Autodesk Fusion 360 part; units mm, degrees
(part 2 of 5)
sketch "Top Projection" plane through (0, 0, 0) normal (0, 0, 1) x (1, 0, 0) in component "Top"
  line L0 (0, 16.095) -> (-1.5613, 16.095)
  arc A0 (-3.175, 17.2242) -> (-1.5613, 16.095) centre (-2.4679, 16.5171) ccw
  line L1 (-3.175, 17.2242) -> (-3.175, 24.7758)
  arc A1 (-1.5613, 25.905) -> (-3.175, 24.7758) centre (-2.4679, 25.4829) ccw
  line L2 (-1.5613, 25.905) -> (0, 25.905)
  line L3 (0, 25.905) -> (0, 36.095)
  line L4 (0, 36.095) -> (-1.5613, 36.095)
  arc A2 (-3.175, 37.2242) -> (-1.5613, 36.095) centre (-2.4679, 36.5171) ccw
  line L5 (-3.175, 37.2242) -> (-3.175, 44.7758)
  arc A3 (-1.5613, 45.905) -> (-3.175, 44.7758) centre (-2.4679, 45.4829) ccw
  line L6 (-1.5613, 45.905) -> (0, 45.905)
  line L7 (0, 45.905) -> (0, 56.095)
  line L8 (0, 56.095) -> (-1.5613, 56.095)
  arc A4 (-3.175, 57.2242) -> (-1.5613, 56.095) centre (-2.4679, 56.5171) ccw
  line L9 (-3.175, 57.2242) -> (-3.175, 64.7758)
  arc A5 (-1.5613, 65.905) -> (-3.175, 64.7758) centre (-2.4679, 65.4829) ccw
  line L10 (-1.5613, 65.905) -> (0, 65.905)
  line L11 (0, 65.905) -> (0, 76.095)
  line L12 (0, 76.095) -> (-1.5613, 76.095)
  arc A6 (-3.175, 77.2242) -> (-1.5613, 76.095) centre (-2.4679, 76.5171) ccw
  line L13 (-3.175, 77.2242) -> (-3.175, 84.7758)
  arc A7 (-1.5613, 85.905) -> (-3.175, 84.7758) centre (-2.4679, 85.4829) ccw
  line L14 (-1.5613, 85.905) -> (0, 85.905)
  line L15 (0, 85.905) -> (0, 96.095)
  line L16 (0, 96.095) -> (-1.5613, 96.095)
  arc A8 (-3.175, 97.2242) -> (-1.5613, 96.095) centre (-2.4679, 96.5171) ccw
  line L17 (-3.175, 97.2242) -> (-3.175, 104.7758)
  arc A9 (-1.5613, 105.905) -> (-3.175, 104.7758) centre (-2.4679, 105.4829) ccw
  line L18 (-1.5613, 105.905) -> (0, 105.905)
  line L19 (0, 105.905) -> (0, 116.095)
  line L20 (0, 116.095) -> (-1.5613, 116.095)
  arc A10 (-3.175, 117.2242) -> (-1.5613, 116.095) centre (-2.4679, 116.5171) ccw
  line L21 (-3.175, 117.2242) -> (-3.175, 124.7758)
  arc A11 (-1.5613, 125.905) -> (-3.175, 124.7758) centre (-2.4679, 125.4829) ccw
  line L22 (-1.5613, 125.905) -> (0, 125.905)
  line L23 (0, 125.905) -> (0, 136.095)
  line L24 (0, 136.095) -> (-1.5613, 136.095)
  arc A12 (-3.175, 137.2242) -> (-1.5613, 136.095) centre (-2.4679, 136.5171) ccw
  line L25 (-3.175, 137.2242) -> (-3.175, 144.7758)
  arc A13 (-1.5613, 145.905) -> (-3.175, 144.7758) centre (-2.4679, 145.4829) ccw
  line L26 (-1.5613, 145.905) -> (0, 145.905)
  line L27 (0, 145.905) -> (0, 156.095)
  line L28 (0, 156.095) -> (-1.5613, 156.095)
  arc A14 (-3.175, 157.2242) -> (-1.5613, 156.095) centre (-2.4679, 156.5171) ccw
  line L29 (-3.175, 157.2242) -> (-3.175, 164.7758)
  arc A15 (-1.5613, 165.905) -> (-3.175, 164.7758) centre (-2.4679, 165.4829) ccw
  line L30 (-1.5613, 165.905) -> (0, 165.905)
  line L31 (0, 165.905) -> (0, 182)
  line L32 (0, 182) -> (-15.095, 182)
  line L33 (-240, 182) -> (-240, 165.905)
  line L34 (-240, 165.905) -> (-238.4387, 165.905)
  arc A16 (-236.825, 164.7758) -> (-238.4387, 165.905) centre (-237.5321, 165.4829) ccw
  line L35 (-236.825, 164.7758) -> (-236.825, 157.2242)
  arc A17 (-238.4387, 156.095) -> (-236.825, 157.2242) centre (-237.5321, 156.5171) ccw
  line L36 (-238.4387, 156.095) -> (-240, 156.095)
  line L37 (-240, 156.095) -> (-240, 145.905)
  line L38 (-240, 145.905) -> (-238.4387, 145.905)
  arc A18 (-236.825, 144.7758) -> (-238.4387, 145.905) centre (-237.5321, 145.4829) ccw
  line L39 (-236.825, 144.7758) -> (-236.825, 137.2242)
  arc A19 (-238.4387, 136.095) -> (-236.825, 137.2242) centre (-237.5321, 136.5171) ccw
  line L40 (-238.4387, 136.095) -> (-240, 136.095)
  line L41 (-240, 136.095) -> (-240, 125.905)
  line L42 (-240, 125.905) -> (-238.4387, 125.905)
  arc A20 (-236.825, 124.7758) -> (-238.4387, 125.905) centre (-237.5321, 125.4829) ccw
  line L43 (-236.825, 124.7758) -> (-236.825, 117.2242)
  arc A21 (-238.4387, 116.095) -> (-236.825, 117.2242) centre (-237.5321, 116.5171) ccw
  line L44 (-238.4387, 116.095) -> (-240, 116.095)
  line L45 (-240, 116.095) -> (-240, 105.905)
  line L46 (-240, 105.905) -> (-238.4387, 105.905)
  arc A22 (-236.825, 104.7758) -> (-238.4387, 105.905) centre (-237.5321, 105.4829) ccw
  line L47 (-236.825, 104.7758) -> (-236.825, 97.2242)
  arc A23 (-238.4387, 96.095) -> (-236.825, 97.2242) centre (-237.5321, 96.5171) ccw
  line L48 (-238.4387, 96.095) -> (-240, 96.095)
  line L49 (-240, 96.095) -> (-240, 85.905)
  line L50 (-240, 85.905) -> (-238.4387, 85.905)
  arc A24 (-236.825, 84.7758) -> (-238.4387, 85.905) centre (-237.5321, 85.4829) ccw
  line L51 (-236.825, 84.7758) -> (-236.825, 77.2242)
  arc A25 (-238.4387, 76.095) -> (-236.825, 77.2242) centre (-237.5321, 76.5171) ccw
  line L52 (-238.4387, 76.095) -> (-240, 76.095)
  line L53 (-240, 76.095) -> (-240, 65.905)
  line L54 (-240, 65.905) -> (-238.4387, 65.905)
  arc A26 (-236.825, 64.7758) -> (-238.4387, 65.905) centre (-237.5321, 65.4829) ccw
  line L55 (-236.825, 64.7758) -> (-236.825, 57.2242)
  arc A27 (-238.4387, 56.095) -> (-236.825, 57.2242) centre (-237.5321, 56.5171) ccw
  line L56 (-238.4387, 56.095) -> (-240, 56.095)
  line L57 (-240, 56.095) -> (-240, 45.905)
  line L58 (-240, 45.905) -> (-238.4387, 45.905)
  arc A28 (-236.825, 44.7758) -> (-238.4387, 45.905) centre (-237.5321, 45.4829) ccw
  line L59 (-236.825, 44.7758) -> (-236.825, 37.2242)
  arc A29 (-238.4387, 36.095) -> (-236.825, 37.2242) centre (-237.5321, 36.5171) ccw
  line L60 (-238.4387, 36.095) -> (-240, 36.095)
  line L61 (-240, 36.095) -> (-240, 25.905)
  line L62 (-240, 25.905) -> (-238.4387, 25.905)
  arc A30 (-236.825, 24.7758) -> (-238.4387, 25.905) centre (-237.5321, 25.4829) ccw
  line L63 (-236.825, 24.7758) -> (-236.825, 17.2242)
  arc A31 (-238.4387, 16.095) -> (-236.825, 17.2242) centre (-237.5321, 16.5171) ccw
  line L64 (-238.4387, 16.095) -> (-240, 16.095)
  line L65 (-240, 16.095) -> (-240, 0)
  line L66 (-240, 0) -> (-224.905, 0)
  line L67 (-224.905, 0) -> (-224.905, 1.5613)
  arc A32 (-223.7758, 3.175) -> (-224.905, 1.5613) centre (-224.4829, 2.4679) ccw
  line L68 (-223.7758, 3.175) -> (-216.2242, 3.175)
  arc A33 (-215.095, 1.5613) -> (-216.2242, 3.175) centre (-215.5171, 2.4679) ccw
  line L69 (-215.095, 1.5613) -> (-215.095, 0)
  line L70 (-215.095, 0) -> (-204.905, 0)
  line L71 (-204.905, 0) -> (-204.905, 1.5613)
  arc A34 (-203.7758, 3.175) -> (-204.905, 1.5613) centre (-204.4829, 2.4679) ccw
  line L72 (-203.7758, 3.175) -> (-196.2242, 3.175)
  arc A35 (-195.095, 1.5613) -> (-196.2242, 3.175) centre (-195.5171, 2.4679) ccw
  line L73 (-195.095, 1.5613) -> (-195.095, 0)
  line L74 (-195.095, 0) -> (-184.905, 0)
  line L75 (-184.905, 0) -> (-184.905, 1.5613)
  arc A36 (-183.7758, 3.175) -> (-184.905, 1.5613) centre (-184.4829, 2.4679) ccw
  line L76 (-183.7758, 3.175) -> (-176.2242, 3.175)
  arc A37 (-175.095, 1.5613) -> (-176.2242, 3.175) centre (-175.5171, 2.4679) ccw
  line L77 (-175.095, 1.5613) -> (-175.095, 0)
  line L78 (-175.095, 0) -> (-164.905, 0)
  line L79 (-164.905, 0) -> (-164.905, 1.5613)
  arc A38 (-163.7758, 3.175) -> (-164.905, 1.5613) centre (-164.4829, 2.4679) ccw
  line L80 (-163.7758, 3.175) -> (-156.2242, 3.175)
  arc A39 (-155.095, 1.5613) -> (-156.2242, 3.175) centre (-155.5171, 2.4679) ccw
  line L81 (-155.095, 1.5613) -> (-155.095, 0)
  line L82 (-155.095, 0) -> (-144.905, 0)
  line L83 (-144.905, 0) -> (-144.905, 1.5613)
  arc A40 (-143.7758, 3.175) -> (-144.905, 1.5613) centre (-144.4829, 2.4679) ccw
  line L84 (-143.7758, 3.175) -> (-136.2242, 3.175)
  arc A41 (-135.095, 1.5613) -> (-136.2242, 3.175) centre (-135.5171, 2.4679) ccw
  line L85 (-135.095, 1.5613) -> (-135.095, 0)
  line L86 (-135.095, 0) -> (-124.905, 0)
  line L87 (-124.905, 0) -> (-124.905, 1.5613)
  arc A42 (-123.7758, 3.175) -> (-124.905, 1.5613) centre (-124.4829, 2.4679) ccw
  line L88 (-123.7758, 3.175) -> (-116.2242, 3.175)
  arc A43 (-115.095, 1.5613) -> (-116.2242, 3.175) centre (-115.5171, 2.4679) ccw
  line L89 (-115.095, 1.5613) -> (-115.095, 0)
  line L90 (-115.095, 0) -> (-104.905, 0)
  line L91 (-104.905, 0) -> (-104.905, 1.5613)
  arc A44 (-103.7758, 3.175) -> (-104.905, 1.5613) centre (-104.4829, 2.4679) ccw
  line L92 (-103.7758, 3.175) -> (-96.2242, 3.175)
  arc A45 (-95.095, 1.5613) -> (-96.2242, 3.175) centre (-95.5171, 2.4679) ccw
  line L93 (-95.095, 1.5613) -> (-95.095, 0)
  line L94 (-95.095, 0) -> (-84.905, 0)
  line L95 (-84.905, 0) -> (-84.905, 1.5613)
  arc A46 (-83.7758, 3.175) -> (-84.905, 1.5613) centre (-84.4829, 2.4679) ccw
  line L96 (-83.7758, 3.175) -> (-76.2242, 3.175)
  arc A47 (-75.095, 1.5613) -> (-76.2242, 3.175) centre (-75.5171, 2.4679) ccw
  line L97 (-75.095, 1.5613) -> (-75.095, 0)
  line L98 (-75.095, 0) -> (-64.905, 0)
  line L99 (-64.905, 0) -> (-64.905, 1.5613)
  arc A48 (-63.7758, 3.175) -> (-64.905, 1.5613) centre (-64.4829, 2.4679) ccw
  line L100 (-63.7758, 3.175) -> (-56.2242, 3.175)
  arc A49 (-55.095, 1.5613) -> (-56.2242, 3.175) centre (-55.5171, 2.4679) ccw
  line L101 (-55.095, 1.5613) -> (-55.095, 0)
  line L102 (-55.095, 0) -> (-44.905, 0)
  line L103 (-44.905, 0) -> (-44.905, 1.5613)
  arc A50 (-43.7758, 3.175) -> (-44.905, 1.5613) centre (-44.4829, 2.4679) ccw
  line L104 (-43.7758, 3.175) -> (-36.2242, 3.175)
  arc A51 (-35.095, 1.5613) -> (-36.2242, 3.175) centre (-35.5171, 2.4679) ccw
  line L105 (-35.095, 1.5613) -> (-35.095, 0)
  line L106 (-35.095, 0) -> (-24.905, 0)
  line L107 (-24.905, 0) -> (-24.905, 1.5613)
  arc A52 (-23.7758, 3.175) -> (-24.905, 1.5613) centre (-24.4829, 2.4679) ccw
  line L108 (-23.7758, 3.175) -> (-16.2242, 3.175)
  arc A53 (-15.095, 1.5613) -> (-16.2242, 3.175) centre (-15.5171, 2.4679) ccw
  line L109 (-15.095, 1.5613) -> (-15.095, 0)
  line L110 (-15.095, 0) -> (0, 0)
  line L111 (0, 0) -> (0, 16.095)
  line L112 (-15.095, 182) -> (-15.095, 180.4387)
  arc A54 (-16.2242, 178.825) -> (-15.095, 180.4387) centre (-15.5171, 179.5321) ccw
  line L113 (-16.2242, 178.825) -> (-23.7758, 178.825)
  arc A55 (-24.905, 180.4387) -> (-23.7758, 178.825) centre (-24.4829, 179.5321) ccw
  line L114 (-24.905, 180.4387) -> (-24.905, 182)
  line L115 (-24.905, 182) -> (-35.095, 182)
  line L116 (-35.095, 182) -> (-35.095, 180.4387)
  arc A56 (-36.2242, 178.825) -> (-35.095, 180.4387) centre (-35.5171, 179.5321) ccw
  line L117 (-36.2242, 178.825) -> (-43.7758, 178.825)
  arc A57 (-44.905, 180.4387) -> (-43.7758, 178.825) centre (-44.4829, 179.5321) ccw
  line L118 (-44.905, 180.4387) -> (-44.905, 182)
  line L119 (-44.905, 182) -> (-55.095, 182)
  line L120 (-55.095, 182) -> (-55.095, 180.4387)
  arc A58 (-56.2242, 178.825) -> (-55.095, 180.4387) centre (-55.5171, 179.5321) ccw
  line L121 (-56.2242, 178.825) -> (-63.7758, 178.825)
  arc A59 (-64.905, 180.4387) -> (-63.7758, 178.825) centre (-64.4829, 179.5321) ccw
  line L122 (-64.905, 180.4387) -> (-64.905, 182)
  line L123 (-64.905, 182) -> (-75.095, 182)
  line L124 (-75.095, 182) -> (-75.095, 180.4387)
  arc A60 (-76.2242, 178.825) -> (-75.095, 180.4387) centre (-75.5171, 179.5321) ccw
  line L125 (-76.2242, 178.825) -> (-83.7758, 178.825)
  arc A61 (-84.905, 180.4387) -> (-83.7758, 178.825) centre (-84.4829, 179.5321) ccw
  line L126 (-84.905, 180.4387) -> (-84.905, 182)
  line L127 (-84.905, 182) -> (-95.095, 182)
  line L128 (-95.095, 182) -> (-95.095, 180.4387)
  arc A62 (-96.2242, 178.825) -> (-95.095, 180.4387) centre (-95.5171, 179.5321) ccw
  line L129 (-96.2242, 178.825) -> (-103.7758, 178.825)
  arc A63 (-104.905, 180.4387) -> (-103.7758, 178.825) centre (-104.4829, 179.5321) ccw
  line L130 (-104.905, 180.4387) -> (-104.905, 182)
  line L131 (-104.905, 182) -> (-115.095, 182)
  line L132 (-115.095, 182) -> (-115.095, 180.4387)
  arc A64 (-116.2242, 178.825) -> (-115.095, 180.4387) centre (-115.5171, 179.5321) ccw
  line L133 (-116.2242, 178.825) -> (-123.7758, 178.825)
  arc A65 (-124.905, 180.4387) -> (-123.7758, 178.825) centre (-124.4829, 179.5321) ccw
  line L134 (-124.905, 180.4387) -> (-124.905, 182)
  line L135 (-124.905, 182) -> (-135.095, 182)
  line L136 (-135.095, 182) -> (-135.095, 180.4387)
  arc A66 (-136.2242, 178.825) -> (-135.095, 180.4387) centre (-135.5171, 179.5321) ccw
  line L137 (-136.2242, 178.825) -> (-143.7758, 178.825)
  arc A67 (-144.905, 180.4387) -> (-143.7758, 178.825) centre (-144.4829, 179.5321) ccw
  line L138 (-144.905, 180.4387) -> (-144.905, 182)
  line L139 (-144.905, 182) -> (-155.095, 182)
  line L140 (-155.095, 182) -> (-155.095, 180.4387)
  arc A68 (-156.2242, 178.825) -> (-155.095, 180.4387) centre (-155.5171, 179.5321) ccw
  line L141 (-156.2242, 178.825) -> (-163.7758, 178.825)
  arc A69 (-164.905, 180.4387) -> (-163.7758, 178.825) centre (-164.4829, 179.5321) ccw
  line L142 (-164.905, 180.4387) -> (-164.905, 182)
  line L143 (-164.905, 182) -> (-175.095, 182)
  line L144 (-175.095, 182) -> (-175.095, 180.4387)
  arc A70 (-176.2242, 178.825) -> (-175.095, 180.4387) centre (-175.5171, 179.5321) ccw
  line L145 (-176.2242, 178.825) -> (-183.7758, 178.825)
  arc A71 (-184.905, 180.4387) -> (-183.7758, 178.825) centre (-184.4829, 179.5321) ccw
  line L146 (-184.905, 180.4387) -> (-184.905, 182)
  line L147 (-184.905, 182) -> (-195.095, 182)
  line L148 (-195.095, 182) -> (-195.095, 180.4387)
  arc A72 (-196.2242, 178.825) -> (-195.095, 180.4387) centre (-195.5171, 179.5321) ccw
  line L149 (-196.2242, 178.825) -> (-203.7758, 178.825)
  arc A73 (-204.905, 180.4387) -> (-203.7758, 178.825) centre (-204.4829, 179.5321) ccw
  line L150 (-204.905, 180.4387) -> (-204.905, 182)
  line L151 (-204.905, 182) -> (-215.095, 182)
  line L152 (-215.095, 182) -> (-215.095, 180.4387)
  arc A74 (-216.2242, 178.825) -> (-215.095, 180.4387) centre (-215.5171, 179.5321) ccw
  line L153 (-216.2242, 178.825) -> (-223.7758, 178.825)
  arc A75 (-224.905, 180.4387) -> (-223.7758, 178.825) centre (-224.4829, 179.5321) ccw
  line L154 (-224.905, 180.4387) -> (-224.905, 182)
  line L155 (-224.905, 182) -> (-240, 182)
sketch "Bottom Projection" plane through (0, 0, 0) normal (0, 0, 1) x (1, 0, 0) in component "Bottom"
  line L0 (0, -158.095) -> (-1.5613, -158.095)
  arc A0 (-1.5613, -158.095) -> (-3.175, -159.2242) centre (-2.4679, -158.5171) ccw
  line L1 (-3.175, -159.2242) -> (-3.175, -166.7758)
  arc A1 (-3.175, -166.7758) -> (-1.5613, -167.905) centre (-2.4679, -167.4829) ccw
  line L2 (-1.5613, -167.905) -> (0, -167.905)
  line L3 (0, -138.095) -> (-1.5613, -138.095)
  arc A2 (-1.5613, -138.095) -> (-3.175, -139.2242) centre (-2.4679, -138.5171) ccw
  line L4 (-3.175, -139.2242) -> (-3.175, -146.7758)
  arc A3 (-3.175, -146.7758) -> (-1.5613, -147.905) centre (-2.4679, -147.4829) ccw
  line L5 (-1.5613, -147.905) -> (0, -147.905)
  line L6 (0, -118.095) -> (-1.5613, -118.095)
  arc A4 (-1.5613, -118.095) -> (-3.175, -119.2242) centre (-2.4679, -118.5171) ccw
  line L7 (-3.175, -119.2242) -> (-3.175, -126.7758)
  arc A5 (-3.175, -126.7758) -> (-1.5613, -127.905) centre (-2.4679, -127.4829) ccw
  line L8 (-1.5613, -127.905) -> (0, -127.905)
  line L9 (0, -98.095) -> (-1.5613, -98.095)
  arc A6 (-1.5613, -98.095) -> (-3.175, -99.2242) centre (-2.4679, -98.5171) ccw
  line L10 (-3.175, -99.2242) -> (-3.175, -106.7758)
  arc A7 (-3.175, -106.7758) -> (-1.5613, -107.905) centre (-2.4679, -107.4829) ccw
  line L11 (-1.5613, -107.905) -> (0, -107.905)
  line L12 (0, -78.095) -> (-1.5613, -78.095)
  arc A8 (-1.5613, -78.095) -> (-3.175, -79.2242) centre (-2.4679, -78.5171) ccw
  line L13 (-3.175, -79.2242) -> (-3.175, -86.7758)
  arc A9 (-3.175, -86.7758) -> (-1.5613, -87.905) centre (-2.4679, -87.4829) ccw
  line L14 (-1.5613, -87.905) -> (0, -87.905)
  line L15 (0, -58.095) -> (-1.5613, -58.095)
  arc A10 (-1.5613, -58.095) -> (-3.175, -59.2242) centre (-2.4679, -58.5171) ccw
  line L16 (-3.175, -59.2242) -> (-3.175, -66.7758)
  arc A11 (-3.175, -66.7758) -> (-1.5613, -67.905) centre (-2.4679, -67.4829) ccw
  line L17 (-1.5613, -67.905) -> (0, -67.905)
  line L18 (0, -38.095) -> (-1.5613, -38.095)
  arc A12 (-1.5613, -38.095) -> (-3.175, -39.2242) centre (-2.4679, -38.5171) ccw
  line L19 (-3.175, -39.2242) -> (-3.175, -46.7758)
  arc A13 (-3.175, -46.7758) -> (-1.5613, -47.905) centre (-2.4679, -47.4829) ccw
  line L20 (-1.5613, -47.905) -> (0, -47.905)
  line L21 (0, -18.095) -> (-1.5613, -18.095)
  arc A14 (-1.5613, -18.095) -> (-3.175, -19.2242) centre (-2.4679, -18.5171) ccw
  line L22 (-3.175, -19.2242) -> (-3.175, -26.7758)
  arc A15 (-3.175, -26.7758) -> (-1.5613, -27.905) centre (-2.4679, -27.4829) ccw
  line L23 (-1.5613, -27.905) -> (0, -27.905)
  line L24 (0, -184) -> (0, -167.905)
  line L25 (0, -158.095) -> (0, -147.905)
  line L26 (0, -138.095) -> (0, -127.905)
  line L27 (0, -118.095) -> (0, -107.905)
  line L28 (0, -98.095) -> (0, -87.905)
  line L29 (0, -78.095) -> (0, -67.905)
  line L30 (0, -58.095) -> (0, -47.905)
  line L31 (0, -38.095) -> (0, -27.905)
  line L32 (0, -18.095) -> (0, -2)
  line L33 (-240, -167.905) -> (-240, -184)
  line L34 (-240, -167.905) -> (-238.4387, -167.905)
  arc A16 (-238.4387, -167.905) -> (-236.825, -166.7758) centre (-237.5321, -167.4829) ccw
  line L35 (-236.825, -166.7758) -> (-236.825, -159.2242)
  arc A17 (-236.825, -159.2242) -> (-238.4387, -158.095) centre (-237.5321, -158.5171) ccw
  line L36 (-238.4387, -158.095) -> (-240, -158.095)
  line L37 (-240, -147.905) -> (-240, -158.095)
  line L38 (-240, -147.905) -> (-238.4387, -147.905)
  arc A18 (-238.4387, -147.905) -> (-236.825, -146.7758) centre (-237.5321, -147.4829) ccw
  line L39 (-236.825, -146.7758) -> (-236.825, -139.2242)
  arc A19 (-236.825, -139.2242) -> (-238.4387, -138.095) centre (-237.5321, -138.5171) ccw
  line L40 (-238.4387, -138.095) -> (-240, -138.095)
  line L41 (-240, -127.905) -> (-240, -138.095)
  line L42 (-240, -127.905) -> (-238.4387, -127.905)
  arc A20 (-238.4387, -127.905) -> (-236.825, -126.7758) centre (-237.5321, -127.4829) ccw
  line L43 (-236.825, -126.7758) -> (-236.825, -119.2242)
  arc A21 (-236.825, -119.2242) -> (-238.4387, -118.095) centre (-237.5321, -118.5171) ccw
  line L44 (-238.4387, -118.095) -> (-240, -118.095)
  line L45 (-240, -107.905) -> (-240, -118.095)
  line L46 (-240, -107.905) -> (-238.4387, -107.905)
  arc A22 (-238.4387, -107.905) -> (-236.825, -106.7758) centre (-237.5321, -107.4829) ccw
  line L47 (-236.825, -106.7758) -> (-236.825, -99.2242)
  arc A23 (-236.825, -99.2242) -> (-238.4387, -98.095) centre (-237.5321, -98.5171) ccw
  line L48 (-238.4387, -98.095) -> (-240, -98.095)
  line L49 (-240, -87.905) -> (-240, -98.095)
  line L50 (-240, -87.905) -> (-238.4387, -87.905)
  arc A24 (-238.4387, -87.905) -> (-236.825, -86.7758) centre (-237.5321, -87.4829) ccw
  line L51 (-236.825, -86.7758) -> (-236.825, -79.2242)
  arc A25 (-236.825, -79.2242) -> (-238.4387, -78.095) centre (-237.5321, -78.5171) ccw
  line L52 (-238.4387, -78.095) -> (-240, -78.095)
  line L53 (-240, -67.905) -> (-240, -78.095)
  line L54 (-240, -67.905) -> (-238.4387, -67.905)
  arc A26 (-238.4387, -67.905) -> (-236.825, -66.7758) centre (-237.5321, -67.4829) ccw
  line L55 (-236.825, -66.7758) -> (-236.825, -59.2242)
  arc A27 (-236.825, -59.2242) -> (-238.4387, -58.095) centre (-237.5321, -58.5171) ccw
  line L56 (-238.4387, -58.095) -> (-240, -58.095)
  line L57 (-240, -47.905) -> (-240, -58.095)
  line L58 (-240, -47.905) -> (-238.4387, -47.905)
  arc A28 (-238.4387, -47.905) -> (-236.825, -46.7758) centre (-237.5321, -47.4829) ccw
  line L59 (-236.825, -46.7758) -> (-236.825, -39.2242)
  arc A29 (-236.825, -39.2242) -> (-238.4387, -38.095) centre (-237.5321, -38.5171) ccw
  line L60 (-238.4387, -38.095) -> (-240, -38.095)
  line L61 (-240, -27.905) -> (-240, -38.095)
  line L62 (-238.4387, -27.905) -> (-240, -27.905)
  arc A30 (-238.4387, -27.905) -> (-236.825, -26.7758) centre (-237.5321, -27.4829) ccw
  line L63 (-236.825, -19.2242) -> (-236.825, -26.7758)
  arc A31 (-236.825, -19.2242) -> (-238.4387, -18.095) centre (-237.5321, -18.5171) ccw
  line L64 (-240, -18.095) -> (-238.4387, -18.095)
  line L65 (-240, -2) -> (-240, -18.095)
  line L66 (-224.905, -2) -> (-224.905, -3.5613)
  arc A32 (-224.905, -3.5613) -> (-223.7758, -5.175) centre (-224.4829, -4.4679) ccw
  line L67 (-223.7758, -5.175) -> (-216.2242, -5.175)
  arc A33 (-216.2242, -5.175) -> (-215.095, -3.5613) centre (-215.5171, -4.4679) ccw
  line L68 (-215.095, -3.5613) -> (-215.095, -2)
  line L69 (-204.905, -2) -> (-215.095, -2)
  line L70 (-204.905, -2) -> (-204.905, -3.5613)
  arc A34 (-204.905, -3.5613) -> (-203.7758, -5.175) centre (-204.4829, -4.4679) ccw
  line L71 (-203.7758, -5.175) -> (-196.2242, -5.175)
  arc A35 (-196.2242, -5.175) -> (-195.095, -3.5613) centre (-195.5171, -4.4679) ccw
  line L72 (-195.095, -3.5613) -> (-195.095, -2)
  line L73 (-184.905, -2) -> (-195.095, -2)
  line L74 (-184.905, -2) -> (-184.905, -3.5613)
  arc A36 (-184.905, -3.5613) -> (-183.7758, -5.175) centre (-184.4829, -4.4679) ccw
  line L75 (-183.7758, -5.175) -> (-176.2242, -5.175)
  arc A37 (-176.2242, -5.175) -> (-175.095, -3.5613) centre (-175.5171, -4.4679) ccw
  line L76 (-175.095, -3.5613) -> (-175.095, -2)
  line L77 (-164.905, -2) -> (-175.095, -2)
  line L78 (-164.905, -2) -> (-164.905, -3.5613)
  arc A38 (-164.905, -3.5613) -> (-163.7758, -5.175) centre (-164.4829, -4.4679) ccw
  line L79 (-163.7758, -5.175) -> (-156.2242, -5.175)
  arc A39 (-156.2242, -5.175) -> (-155.095, -3.5613) centre (-155.5171, -4.4679) ccw
  line L80 (-155.095, -3.5613) -> (-155.095, -2)
  line L81 (-144.905, -2) -> (-155.095, -2)
  line L82 (-144.905, -2) -> (-144.905, -3.5613)
  arc A40 (-144.905, -3.5613) -> (-143.7758, -5.175) centre (-144.4829, -4.4679) ccw
  line L83 (-143.7758, -5.175) -> (-136.2242, -5.175)
  arc A41 (-136.2242, -5.175) -> (-135.095, -3.5613) centre (-135.5171, -4.4679) ccw
  line L84 (-135.095, -3.5613) -> (-135.095, -2)
  line L85 (-124.905, -2) -> (-135.095, -2)
  line L86 (-124.905, -2) -> (-124.905, -3.5613)
  arc A42 (-124.905, -3.5613) -> (-123.7758, -5.175) centre (-124.4829, -4.4679) ccw
  line L87 (-123.7758, -5.175) -> (-116.2242, -5.175)
  arc A43 (-116.2242, -5.175) -> (-115.095, -3.5613) centre (-115.5171, -4.4679) ccw
  line L88 (-115.095, -3.5613) -> (-115.095, -2)
  line L89 (-104.905, -2) -> (-115.095, -2)
  line L90 (-104.905, -2) -> (-104.905, -3.5613)
  arc A44 (-104.905, -3.5613) -> (-103.7758, -5.175) centre (-104.4829, -4.4679) ccw
  line L91 (-103.7758, -5.175) -> (-96.2242, -5.175)
  arc A45 (-96.2242, -5.175) -> (-95.095, -3.5613) centre (-95.5171, -4.4679) ccw
  line L92 (-95.095, -3.5613) -> (-95.095, -2)
  line L93 (-84.905, -2) -> (-95.095, -2)
  line L94 (-84.905, -2) -> (-84.905, -3.5613)
  arc A46 (-84.905, -3.5613) -> (-83.7758, -5.175) centre (-84.4829, -4.4679) ccw
  line L95 (-83.7758, -5.175) -> (-76.2242, -5.175)
  arc A47 (-76.2242, -5.175) -> (-75.095, -3.5613) centre (-75.5171, -4.4679) ccw
  line L96 (-75.095, -3.5613) -> (-75.095, -2)
  line L97 (-64.905, -2) -> (-75.095, -2)
  line L98 (-64.905, -2) -> (-64.905, -3.5613)
  arc A48 (-64.905, -3.5613) -> (-63.7758, -5.175) centre (-64.4829, -4.4679) ccw
  line L99 (-63.7758, -5.175) -> (-56.2242, -5.175)
  arc A49 (-56.2242, -5.175) -> (-55.095, -3.5613) centre (-55.5171, -4.4679) ccw
  line L100 (-55.095, -3.5613) -> (-55.095, -2)
  line L101 (-44.905, -2) -> (-55.095, -2)
  line L102 (-44.905, -2) -> (-44.905, -3.5613)
  arc A50 (-44.905, -3.5613) -> (-43.7758, -5.175) centre (-44.4829, -4.4679) ccw
  line L103 (-43.7758, -5.175) -> (-36.2242, -5.175)
  arc A51 (-36.2242, -5.175) -> (-35.095, -3.5613) centre (-35.5171, -4.4679) ccw
  line L104 (-35.095, -3.5613) -> (-35.095, -2)
  line L105 (-24.905, -2) -> (-35.095, -2)
  line L106 (-24.905, -2) -> (-24.905, -3.5613)
  arc A52 (-24.905, -3.5613) -> (-23.7758, -5.175) centre (-24.4829, -4.4679) ccw
  line L107 (-23.7758, -5.175) -> (-16.2242, -5.175)
  arc A53 (-16.2242, -5.175) -> (-15.095, -3.5613) centre (-15.5171, -4.4679) ccw
  line L108 (-15.095, -3.5613) -> (-15.095, -2)
  line L109 (0, -2) -> (-15.095, -2)
  line L110 (-15.095, -184) -> (-15.095, -182.4387)
  arc A54 (-15.095, -182.4387) -> (-16.2242, -180.825) centre (-15.5171, -181.5321) ccw
  line L111 (-16.2242, -180.825) -> (-23.7758, -180.825)
  arc A55 (-23.7758, -180.825) -> (-24.905, -182.4387) centre (-24.4829, -181.5321) ccw
  line L112 (-24.905, -182.4387) -> (-24.905, -184)
  line L113 (-35.095, -184) -> (-24.905, -184)
  line L114 (-35.095, -184) -> (-35.095, -182.4387)
  arc A56 (-35.095, -182.4387) -> (-36.2242, -180.825) centre (-35.5171, -181.5321) ccw
  line L115 (-36.2242, -180.825) -> (-43.7758, -180.825)
  arc A57 (-43.7758, -180.825) -> (-44.905, -182.4387) centre (-44.4829, -181.5321) ccw
  line L116 (-44.905, -182.4387) -> (-44.905, -184)
  line L117 (-55.095, -184) -> (-44.905, -184)
  line L118 (-55.095, -184) -> (-55.095, -182.4387)
  arc A58 (-55.095, -182.4387) -> (-56.2242, -180.825) centre (-55.5171, -181.5321) ccw
  line L119 (-56.2242, -180.825) -> (-63.7758, -180.825)
  arc A59 (-63.7758, -180.825) -> (-64.905, -182.4387) centre (-64.4829, -181.5321) ccw
  line L120 (-64.905, -182.4387) -> (-64.905, -184)
  line L121 (-75.095, -184) -> (-64.905, -184)
  line L122 (-75.095, -184) -> (-75.095, -182.4387)
  arc A60 (-75.095, -182.4387) -> (-76.2242, -180.825) centre (-75.5171, -181.5321) ccw
  line L123 (-76.2242, -180.825) -> (-83.7758, -180.825)
  arc A61 (-83.7758, -180.825) -> (-84.905, -182.4387) centre (-84.4829, -181.5321) ccw
  line L124 (-84.905, -182.4387) -> (-84.905, -184)
  line L125 (-95.095, -184) -> (-84.905, -184)
  line L126 (-95.095, -184) -> (-95.095, -182.4387)
  arc A62 (-95.095, -182.4387) -> (-96.2242, -180.825) centre (-95.5171, -181.5321) ccw
  line L127 (-96.2242, -180.825) -> (-103.7758, -180.825)
  arc A63 (-103.7758, -180.825) -> (-104.905, -182.4387) centre (-104.4829, -181.5321) ccw
  line L128 (-104.905, -182.4387) -> (-104.905, -184)
  line L129 (-115.095, -184) -> (-104.905, -184)
  line L130 (-115.095, -184) -> (-115.095, -182.4387)
  arc A64 (-115.095, -182.4387) -> (-116.2242, -180.825) centre (-115.5171, -181.5321) ccw
  line L131 (-116.2242, -180.825) -> (-123.7758, -180.825)
  arc A65 (-123.7758, -180.825) -> (-124.905, -182.4387) centre (-124.4829, -181.5321) ccw
  line L132 (-124.905, -182.4387) -> (-124.905, -184)
  line L133 (-135.095, -184) -> (-124.905, -184)
  line L134 (-135.095, -184) -> (-135.095, -182.4387)
  arc A66 (-135.095, -182.4387) -> (-136.2242, -180.825) centre (-135.5171, -181.5321) ccw
  line L135 (-136.2242, -180.825) -> (-143.7758, -180.825)
  arc A67 (-143.7758, -180.825) -> (-144.905, -182.4387) centre (-144.4829, -181.5321) ccw
  line L136 (-144.905, -182.4387) -> (-144.905, -184)
  line L137 (-155.095, -184) -> (-144.905, -184)
  line L138 (-155.095, -184) -> (-155.095, -182.4387)
  arc A68 (-155.095, -182.4387) -> (-156.2242, -180.825) centre (-155.5171, -181.5321) ccw
  line L139 (-156.2242, -180.825) -> (-163.7758, -180.825)
  arc A69 (-163.7758, -180.825) -> (-164.905, -182.4387) centre (-164.4829, -181.5321) ccw
  line L140 (-164.905, -182.4387) -> (-164.905, -184)
  line L141 (-175.095, -184) -> (-164.905, -184)
  line L142 (-175.095, -184) -> (-175.095, -182.4387)
  arc A70 (-175.095, -182.4387) -> (-176.2242, -180.825) centre (-175.5171, -181.5321) ccw
  line L143 (-176.2242, -180.825) -> (-183.7758, -180.825)
  arc A71 (-183.7758, -180.825) -> (-184.905, -182.4387) centre (-184.4829, -181.5321) ccw
  line L144 (-184.905, -182.4387) -> (-184.905, -184)
  line L145 (-195.095, -184) -> (-184.905, -184)
  line L146 (-195.095, -184) -> (-195.095, -182.4387)
  arc A72 (-195.095, -182.4387) -> (-196.2242, -180.825) centre (-195.5171, -181.5321) ccw
  line L147 (-196.2242, -180.825) -> (-203.7758, -180.825)
  arc A73 (-203.7758, -180.825) -> (-204.905, -182.4387) centre (-204.4829, -181.5321) ccw
  line L148 (-204.905, -182.4387) -> (-204.905, -184)
  line L149 (-215.095, -184) -> (-204.905, -184)
  line L150 (-215.095, -184) -> (-215.095, -182.4387)
  arc A74 (-215.095, -182.4387) -> (-216.2242, -180.825) centre (-215.5171, -181.5321) ccw
  line L151 (-216.2242, -180.825) -> (-223.7758, -180.825)
  arc A75 (-223.7758, -180.825) -> (-224.905, -182.4387) centre (-224.4829, -181.5321) ccw
  line L152 (-224.905, -182.4387) -> (-224.905, -184)
  line L153 (-240, -184) -> (-224.905, -184)
  line L154 (-240, -2) -> (-224.905, -2)
  line L155 (-15.095, -184) -> (0, -184)
sketch "Front projection" plane through (0, 0, 0) normal (0, 0, 1) x (1, 0, 0) in component "Front"
  arc A0 (5.175, 6.81) -> (5.175, 8.2242) centre (4.4679, 7.5171) ccw
  line L0 (5.175, 6.81) -> (5.175, 5.175)
  line L1 (5.175, 58.825) -> (5.175, 57.19)
  arc A1 (5.175, 55.7758) -> (5.175, 57.19) centre (4.4679, 56.4829) ccw
  line L2 (5.175, 55.7758) -> (5.175, 48.2242)
  arc A2 (3.5613, 47.095) -> (5.175, 48.2242) centre (4.4679, 47.5171) ccw
  line L3 (3.5613, 47.095) -> (2, 47.095)
  line L4 (2, 36.905) -> (3.5613, 36.905)
  arc A3 (5.175, 35.7758) -> (3.5613, 36.905) centre (4.4679, 36.4829) ccw
  line L5 (5.175, 35.7758) -> (5.175, 28.2242)
  arc A4 (3.5613, 27.095) -> (5.175, 28.2242) centre (4.4679, 27.5171) ccw
  line L6 (3.5613, 27.095) -> (2, 27.095)
  line L7 (2, 16.905) -> (3.5613, 16.905)
  arc A5 (5.175, 15.7758) -> (3.5613, 16.905) centre (4.4679, 16.4829) ccw
  line L8 (5.175, 15.7758) -> (5.175, 8.2242)
  line L9 (15.7758, 58.825) -> (5.175, 58.825)
  line L10 (2, 16.905) -> (2, 27.095)
  arc A6 (238.825, 8.2242) -> (238.825, 6.81) centre (239.5321, 7.5171) ccw
  line L11 (216.905, 62) -> (216.905, 60.4387)
  arc A7 (215.7758, 58.825) -> (216.905, 60.4387) centre (216.4829, 59.5321) ccw
  line L12 (215.7758, 58.825) -> (208.2242, 58.825)
  arc A8 (207.095, 60.4387) -> (208.2242, 58.825) centre (207.5171, 59.5321) ccw
  line L13 (207.095, 60.4387) -> (207.095, 62)
  line L14 (196.905, 62) -> (196.905, 60.4387)
  arc A9 (195.7758, 58.825) -> (196.905, 60.4387) centre (196.4829, 59.5321) ccw
  line L15 (195.7758, 58.825) -> (188.2242, 58.825)
  arc A10 (187.095, 60.4387) -> (188.2242, 58.825) centre (187.5171, 59.5321) ccw
  line L16 (187.095, 60.4387) -> (187.095, 62)
  line L17 (176.905, 62) -> (176.905, 60.4387)
  arc A11 (175.7758, 58.825) -> (176.905, 60.4387) centre (176.4829, 59.5321) ccw
  line L18 (175.7758, 58.825) -> (168.2242, 58.825)
  arc A12 (167.095, 60.4387) -> (168.2242, 58.825) centre (167.5171, 59.5321) ccw
  line L19 (167.095, 60.4387) -> (167.095, 62)
  line L20 (156.905, 62) -> (156.905, 60.4387)
  arc A13 (155.7758, 58.825) -> (156.905, 60.4387) centre (156.4829, 59.5321) ccw
  line L21 (155.7758, 58.825) -> (148.2242, 58.825)
  arc A14 (147.095, 60.4387) -> (148.2242, 58.825) centre (147.5171, 59.5321) ccw
  line L22 (147.095, 60.4387) -> (147.095, 62)
  line L23 (136.905, 62) -> (136.905, 60.4387)
  arc A15 (135.7758, 58.825) -> (136.905, 60.4387) centre (136.4829, 59.5321) ccw
  line L24 (135.7758, 58.825) -> (128.2242, 58.825)
  arc A16 (127.095, 60.4387) -> (128.2242, 58.825) centre (127.5171, 59.5321) ccw
  line L25 (127.095, 60.4387) -> (127.095, 62)
  line L26 (116.905, 62) -> (116.905, 60.4387)
  arc A17 (115.7758, 58.825) -> (116.905, 60.4387) centre (116.4829, 59.5321) ccw
  line L27 (115.7758, 58.825) -> (108.2242, 58.825)
  arc A18 (107.095, 60.4387) -> (108.2242, 58.825) centre (107.5171, 59.5321) ccw
  line L28 (107.095, 60.4387) -> (107.095, 62)
  line L29 (96.905, 62) -> (96.905, 60.4387)
  arc A19 (95.7758, 58.825) -> (96.905, 60.4387) centre (96.4829, 59.5321) ccw
  line L30 (95.7758, 58.825) -> (88.2242, 58.825)
  arc A20 (87.095, 60.4387) -> (88.2242, 58.825) centre (87.5171, 59.5321) ccw
  line L31 (87.095, 60.4387) -> (87.095, 62)
  line L32 (76.905, 62) -> (76.905, 60.4387)
  arc A21 (75.7758, 58.825) -> (76.905, 60.4387) centre (76.4829, 59.5321) ccw
  line L33 (75.7758, 58.825) -> (68.2242, 58.825)
  arc A22 (67.095, 60.4387) -> (68.2242, 58.825) centre (67.5171, 59.5321) ccw
  line L34 (67.095, 60.4387) -> (67.095, 62)
  line L35 (56.905, 62) -> (56.905, 60.4387)
  arc A23 (55.7758, 58.825) -> (56.905, 60.4387) centre (56.4829, 59.5321) ccw
  line L36 (55.7758, 58.825) -> (48.2242, 58.825)
  arc A24 (47.095, 60.4387) -> (48.2242, 58.825) centre (47.5171, 59.5321) ccw
  line L37 (47.095, 60.4387) -> (47.095, 62)
  line L38 (238.825, 58.825) -> (228.2242, 58.825)
  arc A25 (227.095, 60.4387) -> (228.2242, 58.825) centre (227.5171, 59.5321) ccw
  line L39 (227.095, 60.4387) -> (227.095, 62)
  line L40 (36.905, 62) -> (36.905, 60.4387)
  arc A26 (35.7758, 58.825) -> (36.905, 60.4387) centre (36.4829, 59.5321) ccw
  line L41 (35.7758, 58.825) -> (28.2242, 58.825)
  arc A27 (27.095, 60.4387) -> (28.2242, 58.825) centre (27.5171, 59.5321) ccw
  line L42 (27.095, 60.4387) -> (27.095, 62)
  line L43 (16.905, 62) -> (16.905, 60.4387)
  arc A28 (15.7758, 58.825) -> (16.905, 60.4387) centre (16.4829, 59.5321) ccw
  line L44 (238.825, 5.175) -> (238.825, 6.81)
  line L45 (238.825, 58.825) -> (238.825, 57.19)
  line L46 (16.905, 62) -> (27.095, 62)
  line L47 (36.905, 62) -> (47.095, 62)
  line L48 (56.905, 62) -> (67.095, 62)
  line L49 (76.905, 62) -> (87.095, 62)
  line L50 (96.905, 62) -> (107.095, 62)
  line L51 (116.905, 62) -> (127.095, 62)
  line L52 (136.905, 62) -> (147.095, 62)
  line L53 (156.905, 62) -> (167.095, 62)
  line L54 (176.905, 62) -> (187.095, 62)
  line L55 (196.905, 62) -> (207.095, 62)
  line L56 (216.905, 62) -> (227.095, 62)
  arc A29 (238.825, 57.19) -> (238.825, 55.7758) centre (239.5321, 56.4829) ccw
  line L57 (238.825, 55.7758) -> (238.825, 48.2242)
  arc A30 (238.825, 48.2242) -> (240.4387, 47.095) centre (239.5321, 47.5171) ccw
  line L58 (240.4387, 47.095) -> (242, 47.095)
  line L59 (242, 47.095) -> (242, 36.905)
  line L60 (240.4387, 36.905) -> (242, 36.905)
  arc A31 (240.4387, 36.905) -> (238.825, 35.7758) centre (239.5321, 36.4829) ccw
  line L61 (238.825, 28.2242) -> (238.825, 35.7758)
  arc A32 (238.825, 28.2242) -> (240.4387, 27.095) centre (239.5321, 27.5171) ccw
  line L62 (242, 27.095) -> (240.4387, 27.095)
  line L63 (242, 27.095) -> (242, 16.905)
  line L64 (240.4387, 16.905) -> (242, 16.905)
  arc A33 (240.4387, 16.905) -> (238.825, 15.7758) centre (239.5321, 16.4829) ccw
  line L65 (238.825, 8.2242) -> (238.825, 15.7758)
  line L66 (238.825, 5.175) -> (228.2242, 5.175)
  arc A34 (228.2242, 5.175) -> (227.095, 3.5613) centre (227.5171, 4.4679) ccw
  line L67 (227.095, 3.5613) -> (227.095, 2)
  line L68 (227.095, 2) -> (216.905, 2)
  line L69 (216.905, 3.5613) -> (216.905, 2)
  arc A35 (216.905, 3.5613) -> (215.7758, 5.175) centre (216.4829, 4.4679) ccw
  line L70 (208.2242, 5.175) -> (215.7758, 5.175)
  arc A36 (208.2242, 5.175) -> (207.095, 3.5613) centre (207.5171, 4.4679) ccw
  line L71 (207.095, 2) -> (207.095, 3.5613)
  line L72 (207.095, 2) -> (196.905, 2)
  line L73 (196.905, 3.5613) -> (196.905, 2)
  arc A37 (196.905, 3.5613) -> (195.7758, 5.175) centre (196.4829, 4.4679) ccw
  line L74 (188.2242, 5.175) -> (195.7758, 5.175)
  arc A38 (188.2242, 5.175) -> (187.095, 3.5613) centre (187.5171, 4.4679) ccw
  line L75 (187.095, 2) -> (187.095, 3.5613)
  line L76 (187.095, 2) -> (176.905, 2)
  line L77 (176.905, 3.5613) -> (176.905, 2)
  arc A39 (176.905, 3.5613) -> (175.7758, 5.175) centre (176.4829, 4.4679) ccw
  line L78 (168.2242, 5.175) -> (175.7758, 5.175)
  arc A40 (168.2242, 5.175) -> (167.095, 3.5613) centre (167.5171, 4.4679) ccw
  line L79 (167.095, 2) -> (167.095, 3.5613)
  line L80 (167.095, 2) -> (156.905, 2)
  line L81 (156.905, 3.5613) -> (156.905, 2)
  arc A41 (156.905, 3.5613) -> (155.7758, 5.175) centre (156.4829, 4.4679) ccw
  line L82 (148.2242, 5.175) -> (155.7758, 5.175)
  arc A42 (148.2242, 5.175) -> (147.095, 3.5613) centre (147.5171, 4.4679) ccw
  line L83 (147.095, 2) -> (147.095, 3.5613)
  line L84 (147.095, 2) -> (136.905, 2)
  line L85 (136.905, 3.5613) -> (136.905, 2)
  arc A43 (136.905, 3.5613) -> (135.7758, 5.175) centre (136.4829, 4.4679) ccw
  line L86 (128.2242, 5.175) -> (135.7758, 5.175)
  arc A44 (128.2242, 5.175) -> (127.095, 3.5613) centre (127.5171, 4.4679) ccw
  line L87 (127.095, 2) -> (127.095, 3.5613)
  line L88 (127.095, 2) -> (116.905, 2)
  line L89 (116.905, 3.5613) -> (116.905, 2)
  arc A45 (116.905, 3.5613) -> (115.7758, 5.175) centre (116.4829, 4.4679) ccw
  line L90 (108.2242, 5.175) -> (115.7758, 5.175)
  arc A46 (108.2242, 5.175) -> (107.095, 3.5613) centre (107.5171, 4.4679) ccw
  line L91 (107.095, 2) -> (107.095, 3.5613)
  line L92 (107.095, 2) -> (96.905, 2)
  line L93 (96.905, 3.5613) -> (96.905, 2)
  arc A47 (96.905, 3.5613) -> (95.7758, 5.175) centre (96.4829, 4.4679) ccw
  line L94 (88.2242, 5.175) -> (95.7758, 5.175)
  arc A48 (88.2242, 5.175) -> (87.095, 3.5613) centre (87.5171, 4.4679) ccw
  line L95 (87.095, 2) -> (87.095, 3.5613)
  line L96 (87.095, 2) -> (76.905, 2)
  line L97 (76.905, 3.5613) -> (76.905, 2)
  arc A49 (76.905, 3.5613) -> (75.7758, 5.175) centre (76.4829, 4.4679) ccw
  line L98 (68.2242, 5.175) -> (75.7758, 5.175)
  arc A50 (68.2242, 5.175) -> (67.095, 3.5613) centre (67.5171, 4.4679) ccw
  line L99 (67.095, 2) -> (67.095, 3.5613)
  line L100 (67.095, 2) -> (56.905, 2)
  line L101 (56.905, 3.5613) -> (56.905, 2)
  arc A51 (56.905, 3.5613) -> (55.7758, 5.175) centre (56.4829, 4.4679) ccw
  line L102 (48.2242, 5.175) -> (55.7758, 5.175)
  arc A52 (48.2242, 5.175) -> (47.095, 3.5613) centre (47.5171, 4.4679) ccw
  line L103 (47.095, 2) -> (47.095, 3.5613)
  line L104 (47.095, 2) -> (36.905, 2)
  line L105 (36.905, 3.5613) -> (36.905, 2)
  arc A53 (36.905, 3.5613) -> (35.7758, 5.175) centre (36.4829, 4.4679) ccw
  line L106 (28.2242, 5.175) -> (35.7758, 5.175)
  arc A54 (28.2242, 5.175) -> (27.095, 3.5613) centre (27.5171, 4.4679) ccw
  line L107 (27.095, 2) -> (27.095, 3.5613)
  line L108 (27.095, 2) -> (16.905, 2)
  line L109 (16.905, 3.5613) -> (16.905, 2)
  arc A55 (16.905, 3.5613) -> (15.7758, 5.175) centre (16.4829, 4.4679) ccw
  line L110 (5.175, 5.175) -> (15.7758, 5.175)
  line L111 (2, 36.905) -> (2, 47.095)
sketch "Right Projection" plane through (0, 0, 0) normal (0, 0, 1) x (1, 0, 0) in component "Right"
  line L0 (-300.4387, 26.095) -> (-302, 26.095)
  line L1 (-302, 35.905) -> (-300.4387, 35.905)
  arc A0 (-298.825, 34.7758) -> (-300.4387, 35.905) centre (-299.5321, 35.4829) ccw
  line L2 (-298.825, 34.7758) -> (-298.825, 27.2242)
  arc A1 (-300.4387, 26.095) -> (-298.825, 27.2242) centre (-299.5321, 26.5171) ccw
  line L3 (-302, 55.905) -> (-300.4387, 55.905)
  line L4 (-300.4387, 46.095) -> (-302, 46.095)
  arc A2 (-300.4387, 46.095) -> (-298.825, 47.2242) centre (-299.5321, 46.5171) ccw
  line L5 (-298.825, 54.7758) -> (-298.825, 47.2242)
  arc A3 (-298.825, 54.7758) -> (-300.4387, 55.905) centre (-299.5321, 55.4829) ccw
  line L6 (-302, 75.905) -> (-300.4387, 75.905)
  line L7 (-300.4387, 66.095) -> (-302, 66.095)
  arc A4 (-300.4387, 66.095) -> (-298.825, 67.2242) centre (-299.5321, 66.5171) ccw
  line L8 (-298.825, 74.7758) -> (-298.825, 67.2242)
  arc A5 (-298.825, 74.7758) -> (-300.4387, 75.905) centre (-299.5321, 75.4829) ccw
  line L9 (-302, 95.905) -> (-300.4387, 95.905)
  line L10 (-300.4387, 86.095) -> (-302, 86.095)
  arc A6 (-300.4387, 86.095) -> (-298.825, 87.2242) centre (-299.5321, 86.5171) ccw
  line L11 (-298.825, 94.7758) -> (-298.825, 87.2242)
  arc A7 (-298.825, 94.7758) -> (-300.4387, 95.905) centre (-299.5321, 95.4829) ccw
  line L12 (-302, 115.905) -> (-300.4387, 115.905)
  line L13 (-300.4387, 106.095) -> (-302, 106.095)
  arc A8 (-300.4387, 106.095) -> (-298.825, 107.2242) centre (-299.5321, 106.5171) ccw
  line L14 (-298.825, 114.7758) -> (-298.825, 107.2242)
  arc A9 (-298.825, 114.7758) -> (-300.4387, 115.905) centre (-299.5321, 115.4829) ccw
  line L15 (-302, 135.905) -> (-300.4387, 135.905)
  line L16 (-300.4387, 126.095) -> (-302, 126.095)
  arc A10 (-300.4387, 126.095) -> (-298.825, 127.2242) centre (-299.5321, 126.5171) ccw
  line L17 (-298.825, 134.7758) -> (-298.825, 127.2242)
  arc A11 (-298.825, 134.7758) -> (-300.4387, 135.905) centre (-299.5321, 135.4829) ccw
  line L18 (-302, 155.905) -> (-300.4387, 155.905)
  line L19 (-300.4387, 166.095) -> (-302, 166.095)
  arc A12 (-300.4387, 166.095) -> (-298.825, 167.2242) centre (-299.5321, 166.5171) ccw
  line L20 (-298.825, 182) -> (-298.825, 167.2242)
  line L21 (-298.825, 14.7758) -> (-298.825, 0)
  arc A13 (-298.825, 14.7758) -> (-300.4387, 15.905) centre (-299.5321, 15.4829) ccw
  line L22 (-302, 15.905) -> (-300.4387, 15.905)
  line L23 (-300.4387, 146.095) -> (-302, 146.095)
  arc A14 (-300.4387, 146.095) -> (-298.825, 147.2242) centre (-299.5321, 146.5171) ccw
  line L24 (-298.825, 154.7758) -> (-298.825, 147.2242)
  arc A15 (-298.825, 154.7758) -> (-300.4387, 155.905) centre (-299.5321, 155.4829) ccw
  line L25 (-298.825, 0) -> (-286.905, 0)
  line L26 (-302, 26.095) -> (-302, 15.905)
  line L27 (-302, 46.095) -> (-302, 35.905)
  line L28 (-302, 66.095) -> (-302, 55.905)
  line L29 (-302, 86.095) -> (-302, 75.905)
  line L30 (-302, 106.095) -> (-302, 95.905)
  line L31 (-302, 126.095) -> (-302, 115.905)
  line L32 (-302, 146.095) -> (-302, 135.905)
  line L33 (-302, 166.095) -> (-302, 155.905)
  line L34 (-286.905, 182) -> (-298.825, 182)
  line L35 (-286.905, 182) -> (-286.905, 180.4387)
  arc A16 (-286.905, 180.4387) -> (-285.7758, 178.825) centre (-286.4829, 179.5321) ccw
  line L36 (-285.7758, 178.825) -> (-278.2242, 178.825)
  arc A17 (-278.2242, 178.825) -> (-277.095, 180.4387) centre (-277.5171, 179.5321) ccw
  line L37 (-277.095, 180.4387) -> (-277.095, 182)
  line L38 (-266.905, 182) -> (-277.095, 182)
  line L39 (-266.905, 182) -> (-266.905, 180.4387)
  arc A18 (-266.905, 180.4387) -> (-265.7758, 178.825) centre (-266.4829, 179.5321) ccw
  line L40 (-265.7758, 178.825) -> (-258.2242, 178.825)
  arc A19 (-258.2242, 178.825) -> (-257.095, 180.4387) centre (-257.5171, 179.5321) ccw
  line L41 (-257.095, 180.4387) -> (-257.095, 182)
  line L42 (-245.175, 182) -> (-257.095, 182)
  line L43 (-245.175, 182) -> (-245.175, 167.2242)
  arc A20 (-245.175, 167.2242) -> (-243.5613, 166.095) centre (-244.4679, 166.5171) ccw
  line L44 (-243.5613, 166.095) -> (-242, 166.095)
  line L45 (-242, 155.905) -> (-242, 166.095)
  line L46 (-242, 155.905) -> (-243.5613, 155.905)
  arc A21 (-243.5613, 155.905) -> (-245.175, 154.7758) centre (-244.4679, 155.4829) ccw
  line L47 (-245.175, 154.7758) -> (-245.175, 147.2242)
  arc A22 (-245.175, 147.2242) -> (-243.5613, 146.095) centre (-244.4679, 146.5171) ccw
  line L48 (-243.5613, 146.095) -> (-242, 146.095)
  line L49 (-242, 135.905) -> (-242, 146.095)
  line L50 (-242, 135.905) -> (-243.5613, 135.905)
  arc A23 (-243.5613, 135.905) -> (-245.175, 134.7758) centre (-244.4679, 135.4829) ccw
  line L51 (-245.175, 134.7758) -> (-245.175, 127.2242)
  arc A24 (-245.175, 127.2242) -> (-243.5613, 126.095) centre (-244.4679, 126.5171) ccw
  line L52 (-243.5613, 126.095) -> (-242, 126.095)
  line L53 (-242, 115.905) -> (-242, 126.095)
  line L54 (-242, 115.905) -> (-243.5613, 115.905)
  arc A25 (-243.5613, 115.905) -> (-245.175, 114.7758) centre (-244.4679, 115.4829) ccw
  line L55 (-245.175, 114.7758) -> (-245.175, 107.2242)
  arc A26 (-245.175, 107.2242) -> (-243.5613, 106.095) centre (-244.4679, 106.5171) ccw
  line L56 (-243.5613, 106.095) -> (-242, 106.095)
  line L57 (-242, 95.905) -> (-242, 106.095)
  line L58 (-242, 95.905) -> (-243.5613, 95.905)
  arc A27 (-243.5613, 95.905) -> (-245.175, 94.7758) centre (-244.4679, 95.4829) ccw
  line L59 (-245.175, 94.7758) -> (-245.175, 87.2242)
  arc A28 (-245.175, 87.2242) -> (-243.5613, 86.095) centre (-244.4679, 86.5171) ccw
  line L60 (-243.5613, 86.095) -> (-242, 86.095)
  line L61 (-242, 75.905) -> (-242, 86.095)
  line L62 (-242, 75.905) -> (-243.5613, 75.905)
  arc A29 (-243.5613, 75.905) -> (-245.175, 74.7758) centre (-244.4679, 75.4829) ccw
  line L63 (-245.175, 74.7758) -> (-245.175, 67.2242)
  arc A30 (-245.175, 67.2242) -> (-243.5613, 66.095) centre (-244.4679, 66.5171) ccw
  line L64 (-243.5613, 66.095) -> (-242, 66.095)
  line L65 (-242, 55.905) -> (-242, 66.095)
  line L66 (-242, 55.905) -> (-243.5613, 55.905)
  arc A31 (-243.5613, 55.905) -> (-245.175, 54.7758) centre (-244.4679, 55.4829) ccw
  line L67 (-245.175, 54.7758) -> (-245.175, 47.2242)
  arc A32 (-245.175, 47.2242) -> (-243.5613, 46.095) centre (-244.4679, 46.5171) ccw
  line L68 (-243.5613, 46.095) -> (-242, 46.095)
  line L69 (-242, 35.905) -> (-242, 46.095)
  line L70 (-243.5613, 35.905) -> (-242, 35.905)
  arc A33 (-243.5613, 35.905) -> (-245.175, 34.7758) centre (-244.4679, 35.4829) ccw
  line L71 (-245.175, 27.2242) -> (-245.175, 34.7758)
  arc A34 (-245.175, 27.2242) -> (-243.5613, 26.095) centre (-244.4679, 26.5171) ccw
  line L72 (-242, 26.095) -> (-243.5613, 26.095)
  line L73 (-242, 15.905) -> (-242, 26.095)
  line L74 (-243.5613, 15.905) -> (-242, 15.905)
  arc A35 (-243.5613, 15.905) -> (-245.175, 14.7758) centre (-244.4679, 15.4829) ccw
  line L75 (-245.175, 0) -> (-245.175, 14.7758)
  line L76 (-257.095, 0) -> (-245.175, 0)
  line L77 (-257.095, 1.5613) -> (-257.095, 0)
  arc A36 (-257.095, 1.5613) -> (-258.2242, 3.175) centre (-257.5171, 2.4679) ccw
  line L78 (-265.7758, 3.175) -> (-258.2242, 3.175)
  arc A37 (-265.7758, 3.175) -> (-266.905, 1.5613) centre (-266.4829, 2.4679) ccw
  line L79 (-266.905, 0) -> (-266.905, 1.5613)
  line L80 (-277.095, 0) -> (-266.905, 0)
  line L81 (-277.095, 1.5613) -> (-277.095, 0)
  arc A38 (-277.095, 1.5613) -> (-278.2242, 3.175) centre (-277.5171, 2.4679) ccw
  line L82 (-285.7758, 3.175) -> (-278.2242, 3.175)
  arc A39 (-285.7758, 3.175) -> (-286.905, 1.5613) centre (-286.4829, 2.4679) ccw
  line L83 (-286.905, 0) -> (-286.905, 1.5613)